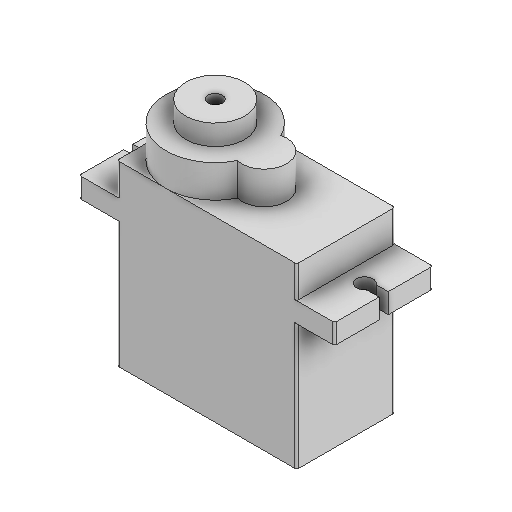
# Autodesk Inventor part: Servo
Saved by Autodesk Inventor 2025.1 (Build 291241020, 241B)
## iProperties
Created: 2024-11-29
Part Number: Servo
Material: Generic
Document SubType Name: Modeling
Designer: alexa
Density: 1 g/cm^3
Appearance: Default
Author: alexa
Autodesk Inventor part; units mm, degrees
ref_plane "YZ Plane" through (0, 0, 0) normal (1, 0, 0) x (0, 1, 0)
sketch "Sketch1" plane through (0, 0, 0) normal (0, 0, 1) x (1, 0, 0)
  line L0 (0, 0) -> (22.4282, 0)
  line L1 (22.4282, 0) -> (22.4282, 22.225)
  line L2 (22.4282, 22.225) -> (0, 22.225)
  line L3 (0, 22.225) -> (0, 0)
  dimension "d0" = 22.4282
  dimension "d1" = 22.225
  constraints: 8 end point, 2 parallel, 1 horizontal, 1 perpendicular
  measures "d0" distance of L0.start L0.end
  measures "d1" distance of L2.end L0.start
extrude "Extrusion1" add sketch "Sketch1" along normal blind 12.2428
ref_plane "Work Plane1" through (0, 18.2372, 0) normal (0, 1, 0) x (1, 0, 0)
sketch "Sketch2" plane through (0, 18.2372, 0) normal (0, 1, 0) x (1, 0, 0)
  line L0 (22.4282, -12.2428) -> (27.1526, -12.2428)
  line L1 (27.1526, 0) -> (22.4282, 0)
  line L2 (22.4282, 0) -> (22.4282, -12.2428)
  arc A0 (25.6304, -5.5499) -> (25.6304, -6.6929) centre (24.7904, -6.1214) ccw
  line L3 (22.4282, 0) -> (22.4282, -12.2428) projected
  line L4 (25.6304, -6.6929) -> (27.1526, -6.6929)
  line L5 (25.6304, -5.5499) -> (27.1526, -5.5499)
  line L6 (27.1526, -12.2428) -> (27.1526, -6.6929)
  line L7 (27.1526, -5.5499) -> (27.1526, 0)
  point P0 (0, 0)
  point P1 (22.4282, -6.1214)
  point P2 (24.7904, 0)
  point P3 (27.1526, -6.1214)
  dimension "d6" = 2.032
  dimension "d23" = 1.143
  dimension "d24" = 0.5715
  dimension "d25" = 4.7244
  constraints: 14 end point, 6 perpendicular, 4 parallel, 2 horizontal alignment, 2 midpoint, 2 point on circle, 2 vertical alignment, 1 centre point, 1 collinear, 1 horizontal
  measures "d6" diameter of A0
  measures "d23" distance between parallel lines of L4 L5
  measures "d24" distance from line of point (27.153, -6.121) L5
  measures "d25" distance between parallel lines of L2 L7
extrude "Extrusion2" add sketch "Sketch2" against normal blind 2.4892
ref_plane "Work Plane2" through (11.2141, 0, 12.2428) normal (1, 0, 0) x (0, 0, -1)
mirror "Mirror1" about plane through (11.2141, 0, 12.2428) normal (1, 0, 0) of "Extrusion2"
sketch "Sketch3" plane through (0, 22.225, 0) normal (0, 1, 0) x (1, 0, 0)
  arc A0 (11.6052, -3.4011) -> (11.6052, -8.8417) centre (6.1214, -6.1214) ccw
  line L0 (22.4282, 0) -> (0, 0) projected
  line L1 (0, 0) -> (0, -12.2428) projected
  line L2 (22.4282, -12.2428) -> (0, -12.2428) projected
  arc A1 (11.6052, -8.8417) -> (11.6052, -3.4011) centre (12.2428, -6.1214) ccw
  dimension "d9" = 5.588
  constraints: 5 point on circle, 3 tangent, 2 centre point, 1 horizontal alignment
  measures "d9" diameter of A1
extrude "Extrusion3" add sketch "Sketch3" along normal blind 4.064 contours A1 A0
sketch "Sketch4" plane through (0, 26.289, 0) normal (0, 1, 0) x (1, 0, 0)
  arc A0 (6.1214, -12.2428) -> (11.6052, -8.8417) centre (6.1214, -6.1214) ccw projected
  circle A1 centre (6.1214, -6.1214) radius 3.6703
  circle A2 centre (6.1214, -6.1214) radius 0.889
  point P0 (0, 0)
  dimension "d12" = 7.3406
  dimension "d15" = 1.778
  constraints: 2 centre point, 2 coincident
  measures "d12" diameter of A1
  measures "d15" diameter of A2
extrude "Extrusion4" add sketch "Sketch4" along normal blind 2.54
sketch "Sketch5" plane through (0, 0, 0) normal (-1, 0, 0) x (0, 0, 1)
  circle A0 centre (4.8514, 4.953) radius 0.635
  circle A1 centre (6.1214, 4.953) radius 0.635
  circle A2 centre (7.3914, 4.953) radius 0.635
  line L0 (4.8514, 4.318) -> (7.3914, 4.318) construction
  line L1 (0, 0) -> (12.2428, 0) projected
  point P0 (6.1214, 0)
  point P1 (6.7564, 4.953)
  point P2 (5.4864, 4.953)
  dimension "d17" = 1.27
  dimension "d18" = 1.27
  dimension "d16" = 1.27
  dimension "d19" = 4.318
  constraints: 2 end point, 2 horizontal alignment, 1 centre point, 1 horizontal, 1 midpoint, 1 vertical alignment, 8 other
  measures "d16" diameter of A1
  measures "d19" distance between parallel lines of L1 L0
extrude "Extrusion5" add sketch "Sketch5" along normal blind 2.54
fillet "Fillet1" radius 0.254 12 edges at (22.4282, 7.874, 0) (22.4282, 20.2311, 0) (22.4282, 20.2311, 12.2428) (22.4282, 7.874, 12.2428) (27.1526, 16.9926, 12.2428) (27.1526, 16.9926, 0) (-4.7244, 16.9926, 0) (-4.7244, 16.9926, 12.2428) (0, 7.874, 12.2428) (0, 7.874, 0) (0, 20.2311, 0) (0, 20.2311, 12.2428)
sketch "Sketch6" plane through (-2.54, 4.953, 4.8514) normal (-1, 0, 0) x (0, 0, 1)
  circle A0 centre (0, 0) radius 0.635 projected
  circle A1 centre (2.54, 0) radius 0.635 projected
  line L0 (-0.635, 0.635) -> (3.175, 0.635)
  line L1 (3.175, 0.635) -> (3.175, -0.635)
  line L2 (3.175, -0.635) -> (-0.635, -0.635)
  line L3 (-0.635, -0.635) -> (-0.635, 0.635)
  circle A2 centre (0, 0) radius 0.635 projected
  circle A3 centre (2.54, 0) radius 0.635 projected
  point P0 (-4.8514, -4.953)
  point P1 (0.635, 0)
  point P2 (1.905, 0)
  constraints: 8 end point, 4 horizontal alignment, 3 horizontal, 2 parallel, 2 vertical, 1 perpendicular
extrude "Extrusion6" add sketch "Sketch6" against normal up to surface (2.54 mm away)
equation "\"d24\" = 0.5 * d23"
equation "\"d17\" = d16"
equation "\"d18\" = d16"
body "Solid1"
